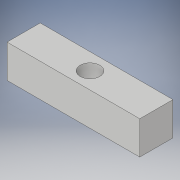
# Autodesk Inventor part: ServoBlock
Saved by Autodesk Inventor 2019 (Build 230136000, 136)
## iProperties
Created: 2019-09-29
Part Number: ServoBlock
Material: Generic
Document SubType Name: Modeling
Designer: james
Density: 1 g/cm^3
Appearance: Default
Author: james
Autodesk Inventor part; units mm, degrees
ref_plane "YZ Plane" through (0, 0, 0) normal (1, 0, 0) x (0, 1, 0)
ref_plane "XZ Plane" through (0, 0, 0) normal (0, 1, 0) x (-1, 0, 0)
ref_plane "XY Plane" through (0, 0, 0) normal (0, 0, 1) x (1, 0, 0)
sketch "Sketch1" plane through (0, 0, 0) normal (1, 0, 0) x (0, 1, 0)
  line L0 (13.7403, 22.0625) -> (-11.6597, 22.0625)
  line L1 (-11.6597, 22.0625) -> (-11.6597, -3.3375)
  line L2 (-11.6597, -3.3375) -> (13.7403, -3.3375)
  line L3 (13.7403, -3.3375) -> (13.7403, 22.0625)
  point P0 (0, 0)
  dimension "d0" = 25.4
  dimension "d1" = 25.4
  constraints: 8 end point, 2 parallel, 1 horizontal, 1 perpendicular
  measures "d0" distance of L0.start L0.end
  measures "d1" distance of L2.end L0.start
extrude "Extrusion1" add sketch "Sketch1" along normal blind 101.6
sketch "Sketch2" plane through (0, 13.7403, 22.0625) normal (0, 1, 0) x (1, 0, 0)
  circle A0 centre (50.8, 12.7) radius 7.5047
  line L0 (0, 25.4) -> (0, 0) projected
  line L1 (0, 25.4) -> (101.6, 25.4) projected
  point P0 (0, 22.0625)
  dimension "d4" = 50.8
  dimension "d5" = 12.7
  constraints: 1 centre point
  measures "d4" distance from line of L0 A0.centre
  measures "d5" distance from line of L1 A0.centre
extrude "Extrusion2" cut sketch "Sketch2" against normal blind 101.6
body "Solid1"
